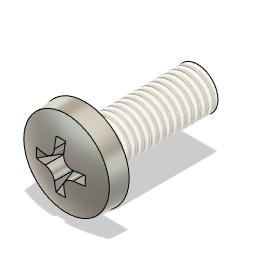
Pineapple case (Autodesk Fusion 360 archive; units mm, degrees)
design "Binding Head Screw JIS B 1111 - M3x8 Steel 4.6 Plain"
description: Binding Head Screw JIS B 1111 - M3x8
part number: BHS JIS B 1111 - M3x8 Steel 4.6 Plain
Autodesk Fusion 360 part; units mm, degrees
(part 1 of 2)
sketch "Sketch1" plane through (0, 0, 0) normal (0, 1, 0) x (1, 0, 0)
  line L0 (0, -1.9) -> (0, 8)
  line L1 (-3.15, 0) -> (-3.0363, -1.3)
  line L2 (-3.15, 0) -> (-1.299, 0)
  arc A0 (-3.0363, -1.3) -> (0, -1.9) centre (0, 6.0824) ccw
  line L3 (0, 8) -> (-1.5, 8)
  line L4 (-1.5, 8) -> (-1.5, 0.94)
  line L5 (-1.5, 0.94) -> (-1.299, 0.19)
  line L6 (-1.299, 0.19) -> (-1.299, 0)
  dimension "d13" = 5
  dimension "d14" = 6.3
  dimension "d18" = 3
  dimension "d23" = 15
  dimension "d53" = 1.9
  dimension "d55" = 7.06
  dimension "d56" = 8
  dimension "d57" = 7.81
  dimension "d60" = 1.3
  constraint vertical L0
  constraint coincident origin L0
  constraint horizontal L2
  constraint coincident origin L2
  constraint coincident L0 A0.end
  constraint coincident L0 A0.centre
  constraint coincident L0.start A0.end
  constraint perpendicular L0 L3
  constraint perpendicular L3 L4
  constraint vertical L6
  constraint coincident L2.end L6.end
  measures "d13" angle of L0 L1
  measures "d23" angle of L4 L5
  measures "d53" distance of L0.start L2
  measures "d55" distance of L3 L4.end
  measures "d56" distance of L2 L3
  measures "d57" distance of L3 L5.end
  measures "d60" distance of L1.end L2
revolve "Revolve1" add sketch "Sketch1" angle 360 about axis through (0, 0, 1.9) along (0, 0, -1) makes body 1
fillet "Fillet2" radius 0.1 1 edges at (-1.2111, 0.4698, 0) on bodies 1
ref_plane "WorkPlane1" through (0, 0, 1.9) normal (0, 0, 1) x (1, 0, 0)
sketch "Sketch2" plane through (0, 0, 1.9) normal (0, 0, 1) x (1, 0, 0)
  line L0 (-1.85, 0) -> (1.85, 0) construction
  line L1 (0, -1.85) -> (0, 1.85) construction
  line L2 (-0.331, 1.85) -> (0.331, 1.85)
  line L3 (0.331, 1.85) -> (0.331, 0.331)
  line L4 (0.331, 0.331) -> (1.85, 0.331)
  line L5 (1.85, 0.331) -> (1.85, -0.331)
  line L6 (1.85, -0.331) -> (0.331, -0.331)
  line L7 (0.331, -0.331) -> (0.331, -1.85)
  line L8 (0.331, -1.85) -> (-0.331, -1.85)
  line L9 (-0.331, -1.85) -> (-0.331, -0.331)
  line L10 (-0.331, -0.331) -> (-1.85, -0.331)
  line L11 (-1.85, -0.331) -> (-1.85, 0.331)
  line L12 (-1.85, 0.331) -> (-0.331, 0.331)
  line L13 (-0.331, 0.331) -> (-0.331, 1.85)
  dimension "d58" = 0.662
  dimension "d59" = 0.662
  dimension "d61" = 3.7
  dimension "d62" = 3.7
  constraint horizontal L0
  constraint vertical L1
  constraint midpoint L0 L1
  constraint midpoint origin L1
  constraint perpendicular L1 L2
  constraint perpendicular L2 L3
  constraint perpendicular L3 L4
  constraint perpendicular L0 L5
  constraint perpendicular L5 L6
  constraint perpendicular L0 L7
  constraint perpendicular L7 L8
  constraint perpendicular L8 L9
  constraint perpendicular L7 L10
  constraint perpendicular L10 L11
  constraint perpendicular L11 L12
  constraint vertical L13
  constraint coincident L9 L12.end
  constraint coincident L3.end L7
  constraint coincident L6 L9.end
  constraint coincident L4 L12.end
  constraint midpoint L0.end L5
  constraint midpoint L1.start L8
  constraint midpoint L1.end L2
  constraint midpoint L0.start L11
  measures "d58" distance of L10 L12
  measures "d59" distance of L3 L13
  measures "d61" distance of L2 L8
  measures "d62" distance of L5 L11
extrude "Extrude1" add sketch "Sketch2" against normal blind 1.53 separate body makes body 2
draft "Draft1" angle -30 neutral plane through (0, 0, 1.9) pull (0, 0, 1) 4 faces at (0.1103, -1.85, 1.39) (-0.1103, 1.85, 1.39) (-1.85, -0.1103, 1.39) (1.85, 0.1103, 1.39) on bodies 2
fillet "Fillet1" radius 0.662 4 edges at (0.331, -0.331, 1.135) (-0.331, -0.331, 1.135) (-0.331, 0.331, 1.135) (0.331, 0.331, 1.135) on bodies 2
combine "Combine1" operation cut target body 1 tool bodies 2
thread "Thread1" "ISO Metric profile 3.0 M3x0.5 M3x0.5 6g" major diameter 2.927 minor diameter 2.3555 pitch 0.5 angle 60 resizes the face on face at (-1.4925, -0.1494, -5.6467) on bodies 1
equation "adsk_nomdia = 3.00 mm"
equation "adsk_nomlen = 8.00 mm"
equation "adsk_headdia = 6.30 mm"
equation "adsk_baseh = 1.30 mm"
equation "adsk_phildia = 3.70 mm"
equation "adsk_midfillet = 0.10 mm"
equation "adsk_thrlen = 7.06 mm"
equation "adsk_phildepth = 1.53 mm"
equation "adsk_thrrun = 0.75 mm"
equation "adsk_thrang = 15.00 deg"
equation "adsk_headang = 5.00 deg"
equation "d13 = adsk_headang"
equation "d14 = adsk_headdia"
equation "adsk_ovalh = 0.60 mm"
equation "d18 = adsk_nomdia"
equation "d23 = adsk_thrang"
equation "d32 = adsk_baseh + adsk_ovalh"
equation "adsk_philwidth = 0.662 mm"
equation "d43 = -adsk_phildepth"
equation "d48 = adsk_philwidth"
equation "d52 = adsk_midfillet"
equation "d53 = adsk_baseh + adsk_ovalh"
equation "d55 = adsk_thrlen"
equation "d56 = adsk_nomlen"
equation "d57 = adsk_thrlen + adsk_thrrun"
equation "d58 = adsk_philwidth"
equation "d59 = adsk_philwidth"
equation "d60 = adsk_baseh"
equation "d61 = adsk_phildia"
equation "d62 = adsk_phildia"

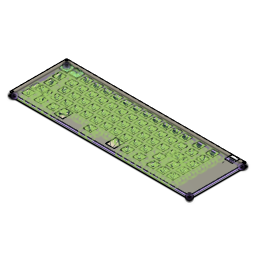
design "Pineappletopcover"
part number: 2025-06-25-20-34-07-285
Autodesk Fusion 360 part; units mm, degrees
sketch "Sketch1" plane through (0, 0, 0) normal (0, 0, 1) x (1, 0, 0)
sketch "Sketch2" plane through (0, 0, 0) normal (0, 0, 1) x (1, 0, 0)
  line L0 (-149.054719, 54.242084) -> (-136.054719, 54.242084)
  line L1 (-149.054719, 40.242084) -> (-136.054719, 40.242084)
  line L2 (-149.554719, 53.742084) -> (-149.554719, 40.742084)
  line L3 (-135.554719, 53.742084) -> (-135.554719, 40.742084)
  arc A0 (-149.054719, 54.242084) -> (-149.554719, 53.742084) centre (-149.054719, 53.742084) ccw
  arc A1 (-135.554719, 53.742084) -> (-136.054719, 54.242084) centre (-136.054719, 53.742084) ccw
  arc A2 (-149.554719, 40.742084) -> (-149.054719, 40.242084) centre (-149.054719, 40.742084) ccw
  arc A3 (-136.054719, 40.242084) -> (-135.554719, 40.742084) centre (-136.054719, 40.742084) ccw
  line L4 (-130.004719, 54.242084) -> (-117.004719, 54.242084)
  line L5 (-130.004719, 40.242084) -> (-117.004719, 40.242084)
  line L6 (-130.504719, 53.742084) -> (-130.504719, 40.742084)
  line L7 (-116.504719, 53.742084) -> (-116.504719, 40.742084)
  arc A4 (-130.004719, 54.242084) -> (-130.504719, 53.742084) centre (-130.004719, 53.742084) ccw
  arc A5 (-116.504719, 53.742084) -> (-117.004719, 54.242084) centre (-117.004719, 53.742084) ccw
  arc A6 (-130.504719, 40.742084) -> (-130.004719, 40.242084) centre (-130.004719, 40.742084) ccw
  arc A7 (-117.004719, 40.242084) -> (-116.504719, 40.742084) centre (-117.004719, 40.742084) ccw
  line L8 (-110.954719, 54.242084) -> (-97.954719, 54.242084)
  line L9 (-110.954719, 40.242084) -> (-97.954719, 40.242084)
  line L10 (-111.454719, 53.742084) -> (-111.454719, 40.742084)
  line L11 (-97.454719, 53.742084) -> (-97.454719, 40.742084)
  arc A8 (-110.954719, 54.242084) -> (-111.454719, 53.742084) centre (-110.954719, 53.742084) ccw
  arc A9 (-97.454719, 53.742084) -> (-97.954719, 54.242084) centre (-97.954719, 53.742084) ccw
  arc A10 (-111.454719, 40.742084) -> (-110.954719, 40.242084) centre (-110.954719, 40.742084) ccw
  arc A11 (-97.954719, 40.242084) -> (-97.454719, 40.742084) centre (-97.954719, 40.742084) ccw
  line L12 (-91.904719, 54.242084) -> (-78.904719, 54.242084)
  line L13 (-91.904719, 40.242084) -> (-78.904719, 40.242084)
  line L14 (-92.404719, 53.742084) -> (-92.404719, 40.742084)
  line L15 (-78.404719, 53.742084) -> (-78.404719, 40.742084)
  arc A12 (-91.904719, 54.242084) -> (-92.404719, 53.742084) centre (-91.904719, 53.742084) ccw
  arc A13 (-78.404719, 53.742084) -> (-78.904719, 54.242084) centre (-78.904719, 53.742084) ccw
  arc A14 (-92.404719, 40.742084) -> (-91.904719, 40.242084) centre (-91.904719, 40.742084) ccw
  arc A15 (-78.904719, 40.242084) -> (-78.404719, 40.742084) centre (-78.904719, 40.742084) ccw
  line L16 (-72.854719, 54.242084) -> (-59.854719, 54.242084)
  line L17 (-72.854719, 40.242084) -> (-59.854719, 40.242084)
  line L18 (-73.354719, 53.742084) -> (-73.354719, 40.742084)
  line L19 (-59.354719, 53.742084) -> (-59.354719, 40.742084)
  arc A16 (-72.854719, 54.242084) -> (-73.354719, 53.742084) centre (-72.854719, 53.742084) ccw
  arc A17 (-59.354719, 53.742084) -> (-59.854719, 54.242084) centre (-59.854719, 53.742084) ccw
  arc A18 (-73.354719, 40.742084) -> (-72.854719, 40.242084) centre (-72.854719, 40.742084) ccw
  arc A19 (-59.854719, 40.242084) -> (-59.354719, 40.742084) centre (-59.854719, 40.742084) ccw
  line L20 (-53.804719, 54.242084) -> (-40.804719, 54.242084)
  line L21 (-53.804719, 40.242084) -> (-40.804719, 40.242084)
  line L22 (-54.304719, 53.742084) -> (-54.304719, 40.742084)
  line L23 (-40.304719, 53.742084) -> (-40.304719, 40.742084)
  arc A20 (-53.804719, 54.242084) -> (-54.304719, 53.742084) centre (-53.804719, 53.742084) ccw
  arc A21 (-40.304719, 53.742084) -> (-40.804719, 54.242084) centre (-40.804719, 53.742084) ccw
  arc A22 (-54.304719, 40.742084) -> (-53.804719, 40.242084) centre (-53.804719, 40.742084) ccw
  arc A23 (-40.804719, 40.242084) -> (-40.304719, 40.742084) centre (-40.804719, 40.742084) ccw
  line L24 (-34.754719, 54.242084) -> (-21.754719, 54.242084)
  line L25 (-34.754719, 40.242084) -> (-21.754719, 40.242084)
  line L26 (-35.254719, 53.742084) -> (-35.254719, 40.742084)
  line L27 (-21.254719, 53.742084) -> (-21.254719, 40.742084)
  arc A24 (-34.754719, 54.242084) -> (-35.254719, 53.742084) centre (-34.754719, 53.742084) ccw
  arc A25 (-21.254719, 53.742084) -> (-21.754719, 54.242084) centre (-21.754719, 53.742084) ccw
  arc A26 (-35.254719, 40.742084) -> (-34.754719, 40.242084) centre (-34.754719, 40.742084) ccw
  arc A27 (-21.754719, 40.242084) -> (-21.254719, 40.742084) centre (-21.754719, 40.742084) ccw
  line L28 (-15.704719, 54.242084) -> (-2.704719, 54.242084)
  line L29 (-15.704719, 40.242084) -> (-2.704719, 40.242084)
  line L30 (-16.204719, 53.742084) -> (-16.204719, 40.742084)
  line L31 (-2.204719, 53.742084) -> (-2.204719, 40.742084)
  arc A28 (-15.704719, 54.242084) -> (-16.204719, 53.742084) centre (-15.704719, 53.742084) ccw
  arc A29 (-2.204719, 53.742084) -> (-2.704719, 54.242084) centre (-2.704719, 53.742084) ccw
  arc A30 (-16.204719, 40.742084) -> (-15.704719, 40.242084) centre (-15.704719, 40.742084) ccw
  arc A31 (-2.704719, 40.242084) -> (-2.204719, 40.742084) centre (-2.704719, 40.742084) ccw
  line L32 (3.345281, 54.242084) -> (16.345281, 54.242084)
  line L33 (3.345281, 40.242084) -> (16.345281, 40.242084)
  line L34 (2.845281, 53.742084) -> (2.845281, 40.742084)
  line L35 (16.845281, 53.742084) -> (16.845281, 40.742084)
  arc A32 (3.345281, 54.242084) -> (2.845281, 53.742084) centre (3.345281, 53.742084) ccw
  arc A33 (16.845281, 53.742084) -> (16.345281, 54.242084) centre (16.345281, 53.742084) ccw
  arc A34 (2.845281, 40.742084) -> (3.345281, 40.242084) centre (3.345281, 40.742084) ccw
  arc A35 (16.345281, 40.242084) -> (16.845281, 40.742084) centre (16.345281, 40.742084) ccw
  line L36 (22.395281, 54.242084) -> (35.395281, 54.242084)
  line L37 (22.395281, 40.242084) -> (35.395281, 40.242084)
  line L38 (21.895281, 53.742084) -> (21.895281, 40.742084)
  line L39 (35.895281, 53.742084) -> (35.895281, 40.742084)
  arc A36 (22.395281, 54.242084) -> (21.895281, 53.742084) centre (22.395281, 53.742084) ccw
  arc A37 (35.895281, 53.742084) -> (35.395281, 54.242084) centre (35.395281, 53.742084) ccw
  arc A38 (21.895281, 40.742084) -> (22.395281, 40.242084) centre (22.395281, 40.742084) ccw
  arc A39 (35.395281, 40.242084) -> (35.895281, 40.742084) centre (35.395281, 40.742084) ccw
  line L40 (41.445281, 54.242084) -> (54.445281, 54.242084)
  line L41 (41.445281, 40.242084) -> (54.445281, 40.242084)
  line L42 (40.945281, 53.742084) -> (40.945281, 40.742084)
  line L43 (54.945281, 53.742084) -> (54.945281, 40.742084)
  arc A40 (41.445281, 54.242084) -> (40.945281, 53.742084) centre (41.445281, 53.742084) ccw
  arc A41 (54.945281, 53.742084) -> (54.445281, 54.242084) centre (54.445281, 53.742084) ccw
  arc A42 (40.945281, 40.742084) -> (41.445281, 40.242084) centre (41.445281, 40.742084) ccw
  arc A43 (54.445281, 40.242084) -> (54.945281, 40.742084) centre (54.445281, 40.742084) ccw
  line L44 (60.495281, 54.242084) -> (73.495281, 54.242084)
  line L45 (60.495281, 40.242084) -> (73.495281, 40.242084)
  line L46 (59.995281, 53.742084) -> (59.995281, 40.742084)
  line L47 (73.995281, 53.742084) -> (73.995281, 40.742084)
  arc A44 (60.495281, 54.242084) -> (59.995281, 53.742084) centre (60.495281, 53.742084) ccw
  arc A45 (73.995281, 53.742084) -> (73.495281, 54.242084) centre (73.495281, 53.742084) ccw
  arc A46 (59.995281, 40.742084) -> (60.495281, 40.242084) centre (60.495281, 40.742084) ccw
  arc A47 (73.495281, 40.242084) -> (73.995281, 40.742084) centre (73.495281, 40.742084) ccw
  line L48 (79.545281, 54.242084) -> (92.545281, 54.242084)
  line L49 (79.545281, 40.242084) -> (92.545281, 40.242084)
  line L50 (79.045281, 53.742084) -> (79.045281, 40.742084)
  line L51 (93.045281, 53.742084) -> (93.045281, 40.742084)
  arc A48 (79.545281, 54.242084) -> (79.045281, 53.742084) centre (79.545281, 53.742084) ccw
  arc A49 (93.045281, 53.742084) -> (92.545281, 54.242084) centre (92.545281, 53.742084) ccw
  arc A50 (79.045281, 40.742084) -> (79.545281, 40.242084) centre (79.545281, 40.742084) ccw
  arc A51 (92.545281, 40.242084) -> (93.045281, 40.742084) centre (92.545281, 40.742084) ccw
  line L52 (105.739031, 54.242084) -> (118.739031, 54.242084)
  line L53 (105.739031, 40.242084) -> (118.739031, 40.242084)
  line L54 (105.239031, 53.742084) -> (105.239031, 40.742084)
  line L55 (119.239031, 53.742084) -> (119.239031, 40.742084)
  arc A52 (105.739031, 54.242084) -> (105.239031, 53.742084) centre (105.739031, 53.742084) ccw
  arc A53 (119.239031, 53.742084) -> (118.739031, 54.242084) centre (118.739031, 53.742084) ccw
  arc A54 (105.239031, 40.742084) -> (105.739031, 40.242084) centre (105.739031, 40.742084) ccw
  arc A55 (118.739031, 40.242084) -> (119.239031, 40.742084) centre (118.739031, 40.742084) ccw
  line L56 (131.932781, 54.242084) -> (144.932781, 54.242084)
  line L57 (131.932781, 40.242084) -> (144.932781, 40.242084)
  line L58 (131.432781, 53.742084) -> (131.432781, 40.742084)
  line L59 (145.432781, 53.742084) -> (145.432781, 40.742084)
  arc A56 (131.932781, 54.242084) -> (131.432781, 53.742084) centre (131.932781, 53.742084) ccw
  arc A57 (145.432781, 53.742084) -> (144.932781, 54.242084) centre (144.932781, 53.742084) ccw
  arc A58 (131.432781, 40.742084) -> (131.932781, 40.242084) centre (131.932781, 40.742084) ccw
  arc A59 (144.932781, 40.242084) -> (145.432781, 40.742084) centre (144.932781, 40.742084) ccw
  line L60 (-144.292219, 35.192084) -> (-131.292219, 35.192084)
  line L61 (-144.292219, 21.192084) -> (-131.292219, 21.192084)
  line L62 (-144.792219, 34.692084) -> (-144.792219, 21.692084)
  line L63 (-130.792219, 34.692084) -> (-130.792219, 21.692084)
  arc A60 (-144.292219, 35.192084) -> (-144.792219, 34.692084) centre (-144.292219, 34.692084) ccw
  arc A61 (-130.792219, 34.692084) -> (-131.292219, 35.192084) centre (-131.292219, 34.692084) ccw
  arc A62 (-144.792219, 21.692084) -> (-144.292219, 21.192084) centre (-144.292219, 21.692084) ccw
  arc A63 (-131.292219, 21.192084) -> (-130.792219, 21.692084) centre (-131.292219, 21.692084) ccw
  line L64 (-120.479719, 35.192084) -> (-107.479719, 35.192084)
  line L65 (-120.479719, 21.192084) -> (-107.479719, 21.192084)
  line L66 (-120.979719, 34.692084) -> (-120.979719, 21.692084)
  line L67 (-106.979719, 34.692084) -> (-106.979719, 21.692084)
  arc A64 (-120.479719, 35.192084) -> (-120.979719, 34.692084) centre (-120.479719, 34.692084) ccw
  arc A65 (-106.979719, 34.692084) -> (-107.479719, 35.192084) centre (-107.479719, 34.692084) ccw
  arc A66 (-120.979719, 21.692084) -> (-120.479719, 21.192084) centre (-120.479719, 21.692084) ccw
  arc A67 (-107.479719, 21.192084) -> (-106.979719, 21.692084) centre (-107.479719, 21.692084) ccw
  line L68 (-101.429719, 35.192084) -> (-88.429719, 35.192084)
  line L69 (-101.429719, 21.192084) -> (-88.429719, 21.192084)
  line L70 (-101.929719, 34.692084) -> (-101.929719, 21.692084)
  line L71 (-87.929719, 34.692084) -> (-87.929719, 21.692084)
  arc A68 (-101.429719, 35.192084) -> (-101.929719, 34.692084) centre (-101.429719, 34.692084) ccw
  arc A69 (-87.929719, 34.692084) -> (-88.429719, 35.192084) centre (-88.429719, 34.692084) ccw
  arc A70 (-101.929719, 21.692084) -> (-101.429719, 21.192084) centre (-101.429719, 21.692084) ccw
  arc A71 (-88.429719, 21.192084) -> (-87.929719, 21.692084) centre (-88.429719, 21.692084) ccw
  line L72 (-82.379719, 35.192084) -> (-69.379719, 35.192084)
  line L73 (-82.379719, 21.192084) -> (-69.379719, 21.192084)
  line L74 (-82.879719, 34.692084) -> (-82.879719, 21.692084)
  line L75 (-68.879719, 34.692084) -> (-68.879719, 21.692084)
  arc A72 (-82.379719, 35.192084) -> (-82.879719, 34.692084) centre (-82.379719, 34.692084) ccw
  arc A73 (-68.879719, 34.692084) -> (-69.379719, 35.192084) centre (-69.379719, 34.692084) ccw
  arc A74 (-82.879719, 21.692084) -> (-82.379719, 21.192084) centre (-82.379719, 21.692084) ccw
  arc A75 (-69.379719, 21.192084) -> (-68.879719, 21.692084) centre (-69.379719, 21.692084) ccw
  line L76 (-63.329719, 35.192084) -> (-50.329719, 35.192084)
  line L77 (-63.329719, 21.192084) -> (-50.329719, 21.192084)
  line L78 (-63.829719, 34.692084) -> (-63.829719, 21.692084)
  line L79 (-49.829719, 34.692084) -> (-49.829719, 21.692084)
  arc A76 (-63.329719, 35.192084) -> (-63.829719, 34.692084) centre (-63.329719, 34.692084) ccw
  arc A77 (-49.829719, 34.692084) -> (-50.329719, 35.192084) centre (-50.329719, 34.692084) ccw
  arc A78 (-63.829719, 21.692084) -> (-63.329719, 21.192084) centre (-63.329719, 21.692084) ccw
  arc A79 (-50.329719, 21.192084) -> (-49.829719, 21.692084) centre (-50.329719, 21.692084) ccw
  line L80 (-44.279719, 35.192084) -> (-31.279719, 35.192084)
  line L81 (-44.279719, 21.192084) -> (-31.279719, 21.192084)
  line L82 (-44.779719, 34.692084) -> (-44.779719, 21.692084)
  line L83 (-30.779719, 34.692084) -> (-30.779719, 21.692084)
  arc A80 (-44.279719, 35.192084) -> (-44.779719, 34.692084) centre (-44.279719, 34.692084) ccw
  arc A81 (-30.779719, 34.692084) -> (-31.279719, 35.192084) centre (-31.279719, 34.692084) ccw
  arc A82 (-44.779719, 21.692084) -> (-44.279719, 21.192084) centre (-44.279719, 21.692084) ccw
  arc A83 (-31.279719, 21.192084) -> (-30.779719, 21.692084) centre (-31.279719, 21.692084) ccw
  line L84 (-25.229719, 35.192084) -> (-12.229719, 35.192084)
  line L85 (-25.229719, 21.192084) -> (-12.229719, 21.192084)
  line L86 (-25.729719, 34.692084) -> (-25.729719, 21.692084)
  line L87 (-11.729719, 34.692084) -> (-11.729719, 21.692084)
  arc A84 (-25.229719, 35.192084) -> (-25.729719, 34.692084) centre (-25.229719, 34.692084) ccw
  arc A85 (-11.729719, 34.692084) -> (-12.229719, 35.192084) centre (-12.229719, 34.692084) ccw
  arc A86 (-25.729719, 21.692084) -> (-25.229719, 21.192084) centre (-25.229719, 21.692084) ccw
  arc A87 (-12.229719, 21.192084) -> (-11.729719, 21.692084) centre (-12.229719, 21.692084) ccw
  line L88 (-6.179719, 35.192084) -> (6.820281, 35.192084)
  line L89 (-6.179719, 21.192084) -> (6.820281, 21.192084)
  line L90 (-6.679719, 34.692084) -> (-6.679719, 21.692084)
  line L91 (7.320281, 34.692084) -> (7.320281, 21.692084)
  arc A88 (-6.179719, 35.192084) -> (-6.679719, 34.692084) centre (-6.179719, 34.692084) ccw
  arc A89 (7.320281, 34.692084) -> (6.820281, 35.192084) centre (6.820281, 34.692084) ccw
  arc A90 (-6.679719, 21.692084) -> (-6.179719, 21.192084) centre (-6.179719, 21.692084) ccw
  arc A91 (6.820281, 21.192084) -> (7.320281, 21.692084) centre (6.820281, 21.692084) ccw
  line L92 (12.870281, 35.192084) -> (25.870281, 35.192084)
  line L93 (12.870281, 21.192084) -> (25.870281, 21.192084)
  line L94 (12.370281, 34.692084) -> (12.370281, 21.692084)
  line L95 (26.370281, 34.692084) -> (26.370281, 21.692084)
  arc A92 (12.870281, 35.192084) -> (12.370281, 34.692084) centre (12.870281, 34.692084) ccw
  arc A93 (26.370281, 34.692084) -> (25.870281, 35.192084) centre (25.870281, 34.692084) ccw
  arc A94 (12.370281, 21.692084) -> (12.870281, 21.192084) centre (12.870281, 21.692084) ccw
  arc A95 (25.870281, 21.192084) -> (26.370281, 21.692084) centre (25.870281, 21.692084) ccw
  line L96 (31.920281, 35.192084) -> (44.920281, 35.192084)
  line L97 (31.920281, 21.192084) -> (44.920281, 21.192084)
  line L98 (31.420281, 34.692084) -> (31.420281, 21.692084)
  line L99 (45.420281, 34.692084) -> (45.420281, 21.692084)
  arc A96 (31.920281, 35.192084) -> (31.420281, 34.692084) centre (31.920281, 34.692084) ccw
  arc A97 (45.420281, 34.692084) -> (44.920281, 35.192084) centre (44.920281, 34.692084) ccw
  arc A98 (31.420281, 21.692084) -> (31.920281, 21.192084) centre (31.920281, 21.692084) ccw
  arc A99 (44.920281, 21.192084) -> (45.420281, 21.692084) centre (44.920281, 21.692084) ccw
  line L100 (50.970281, 35.192084) -> (63.970281, 35.192084)
  line L101 (50.970281, 21.192084) -> (63.970281, 21.192084)
  line L102 (50.470281, 34.692084) -> (50.470281, 21.692084)
  line L103 (64.470281, 34.692084) -> (64.470281, 21.692084)
  arc A100 (50.970281, 35.192084) -> (50.470281, 34.692084) centre (50.970281, 34.692084) ccw
  arc A101 (64.470281, 34.692084) -> (63.970281, 35.192084) centre (63.970281, 34.692084) ccw
  arc A102 (50.470281, 21.692084) -> (50.970281, 21.192084) centre (50.970281, 21.692084) ccw
  arc A103 (63.970281, 21.192084) -> (64.470281, 21.692084) centre (63.970281, 21.692084) ccw
  line L104 (70.020281, 35.192084) -> (83.020281, 35.192084)
  line L105 (70.020281, 21.192084) -> (83.020281, 21.192084)
  line L106 (69.520281, 34.692084) -> (69.520281, 21.692084)
  line L107 (83.520281, 34.692084) -> (83.520281, 21.692084)
  arc A104 (70.020281, 35.192084) -> (69.520281, 34.692084) centre (70.020281, 34.692084) ccw
  arc A105 (83.520281, 34.692084) -> (83.020281, 35.192084) centre (83.020281, 34.692084) ccw
  arc A106 (69.520281, 21.692084) -> (70.020281, 21.192084) centre (70.020281, 21.692084) ccw
  arc A107 (83.020281, 21.192084) -> (83.520281, 21.692084) centre (83.020281, 21.692084) ccw
  line L108 (89.070281, 35.192084) -> (102.070281, 35.192084)
  line L109 (89.070281, 21.192084) -> (102.070281, 21.192084)
  line L110 (88.570281, 34.692084) -> (88.570281, 21.692084)
  line L111 (102.570281, 34.692084) -> (102.570281, 21.692084)
  arc A108 (89.070281, 35.192084) -> (88.570281, 34.692084) centre (89.070281, 34.692084) ccw
  arc A109 (102.570281, 34.692084) -> (102.070281, 35.192084) centre (102.070281, 34.692084) ccw
  arc A110 (88.570281, 21.692084) -> (89.070281, 21.192084) centre (89.070281, 21.692084) ccw
  arc A111 (102.070281, 21.192084) -> (102.570281, 21.692084) centre (102.070281, 21.692084) ccw
  line L112 (110.501531, 35.192084) -> (123.501531, 35.192084)
  line L113 (110.501531, 21.192084) -> (123.501531, 21.192084)
  line L114 (110.001531, 34.692084) -> (110.001531, 21.692084)
  line L115 (124.001531, 34.692084) -> (124.001531, 21.692084)
  arc A112 (110.501531, 35.192084) -> (110.001531, 34.692084) centre (110.501531, 34.692084) ccw
  arc A113 (124.001531, 34.692084) -> (123.501531, 35.192084) centre (123.501531, 34.692084) ccw
  arc A114 (110.001531, 21.692084) -> (110.501531, 21.192084) centre (110.501531, 21.692084) ccw
  arc A115 (123.501531, 21.192084) -> (124.001531, 21.692084) centre (123.501531, 21.692084) ccw
  line L116 (131.932781, 35.192084) -> (144.932781, 35.192084)
  line L117 (131.932781, 21.192084) -> (144.932781, 21.192084)
  line L118 (131.432781, 34.692084) -> (131.432781, 21.692084)
  line L119 (145.432781, 34.692084) -> (145.432781, 21.692084)
  arc A116 (131.932781, 35.192084) -> (131.432781, 34.692084) centre (131.932781, 34.692084) ccw
  arc A117 (145.432781, 34.692084) -> (144.932781, 35.192084) centre (144.932781, 34.692084) ccw
  arc A118 (131.432781, 21.692084) -> (131.932781, 21.192084) centre (131.932781, 21.692084) ccw
  arc A119 (144.932781, 21.192084) -> (145.432781, 21.692084) centre (144.932781, 21.692084) ccw
  line L120 (-141.910969, 16.142084) -> (-128.910969, 16.142084)
  line L121 (-141.910969, 2.142084) -> (-128.910969, 2.142084)
  line L122 (-142.410969, 15.642084) -> (-142.410969, 2.642084)
  line L123 (-128.410969, 15.642084) -> (-128.410969, 2.642084)
  arc A120 (-141.910969, 16.142084) -> (-142.410969, 15.642084) centre (-141.910969, 15.642084) ccw
  arc A121 (-128.410969, 15.642084) -> (-128.910969, 16.142084) centre (-128.910969, 15.642084) ccw
  arc A122 (-142.410969, 2.642084) -> (-141.910969, 2.142084) centre (-141.910969, 2.642084) ccw
  arc A123 (-128.910969, 2.142084) -> (-128.410969, 2.642084) centre (-128.910969, 2.642084) ccw
  line L124 (-115.717219, 16.142084) -> (-102.717219, 16.142084)
  line L125 (-115.717219, 2.142084) -> (-102.717219, 2.142084)
  line L126 (-116.217219, 15.642084) -> (-116.217219, 2.642084)
  line L127 (-102.217219, 15.642084) -> (-102.217219, 2.642084)
  arc A124 (-115.717219, 16.142084) -> (-116.217219, 15.642084) centre (-115.717219, 15.642084) ccw
  arc A125 (-102.217219, 15.642084) -> (-102.717219, 16.142084) centre (-102.717219, 15.642084) ccw
  arc A126 (-116.217219, 2.642084) -> (-115.717219, 2.142084) centre (-115.717219, 2.642084) ccw
  arc A127 (-102.717219, 2.142084) -> (-102.217219, 2.642084) centre (-102.717219, 2.642084) ccw
  line L128 (-96.667219, 16.142084) -> (-83.667219, 16.142084)
  line L129 (-96.667219, 2.142084) -> (-83.667219, 2.142084)
  line L130 (-97.167219, 15.642084) -> (-97.167219, 2.642084)
  line L131 (-83.167219, 15.642084) -> (-83.167219, 2.642084)
  arc A128 (-96.667219, 16.142084) -> (-97.167219, 15.642084) centre (-96.667219, 15.642084) ccw
  arc A129 (-83.167219, 15.642084) -> (-83.667219, 16.142084) centre (-83.667219, 15.642084) ccw
  arc A130 (-97.167219, 2.642084) -> (-96.667219, 2.142084) centre (-96.667219, 2.642084) ccw
  arc A131 (-83.667219, 2.142084) -> (-83.167219, 2.642084) centre (-83.667219, 2.642084) ccw
  line L132 (-77.617219, 16.142084) -> (-64.617219, 16.142084)
  line L133 (-77.617219, 2.142084) -> (-64.617219, 2.142084)
  line L134 (-78.117219, 15.642084) -> (-78.117219, 2.642084)
  line L135 (-64.117219, 15.642084) -> (-64.117219, 2.642084)
  arc A132 (-77.617219, 16.142084) -> (-78.117219, 15.642084) centre (-77.617219, 15.642084) ccw
  arc A133 (-64.117219, 15.642084) -> (-64.617219, 16.142084) centre (-64.617219, 15.642084) ccw
  arc A134 (-78.117219, 2.642084) -> (-77.617219, 2.142084) centre (-77.617219, 2.642084) ccw
  arc A135 (-64.617219, 2.142084) -> (-64.117219, 2.642084) centre (-64.617219, 2.642084) ccw
  line L136 (-58.567219, 16.142084) -> (-45.567219, 16.142084)
  line L137 (-58.567219, 2.142084) -> (-45.567219, 2.142084)
  line L138 (-59.067219, 15.642084) -> (-59.067219, 2.642084)
  line L139 (-45.067219, 15.642084) -> (-45.067219, 2.642084)
  arc A136 (-58.567219, 16.142084) -> (-59.067219, 15.642084) centre (-58.567219, 15.642084) ccw
  arc A137 (-45.067219, 15.642084) -> (-45.567219, 16.142084) centre (-45.567219, 15.642084) ccw
  arc A138 (-59.067219, 2.642084) -> (-58.567219, 2.142084) centre (-58.567219, 2.642084) ccw
  arc A139 (-45.567219, 2.142084) -> (-45.067219, 2.642084) centre (-45.567219, 2.642084) ccw
  line L140 (-39.517219, 16.142084) -> (-26.517219, 16.142084)
  line L141 (-39.517219, 2.142084) -> (-26.517219, 2.142084)
  line L142 (-40.017219, 15.642084) -> (-40.017219, 2.642084)
  line L143 (-26.017219, 15.642084) -> (-26.017219, 2.642084)
  arc A140 (-39.517219, 16.142084) -> (-40.017219, 15.642084) centre (-39.517219, 15.642084) ccw
  arc A141 (-26.017219, 15.642084) -> (-26.517219, 16.142084) centre (-26.517219, 15.642084) ccw
  arc A142 (-40.017219, 2.642084) -> (-39.517219, 2.142084) centre (-39.517219, 2.642084) ccw
  arc A143 (-26.517219, 2.142084) -> (-26.017219, 2.642084) centre (-26.517219, 2.642084) ccw
  line L144 (-20.467219, 16.142084) -> (-7.467219, 16.142084)
  line L145 (-20.467219, 2.142084) -> (-7.467219, 2.142084)
  line L146 (-20.967219, 15.642084) -> (-20.967219, 2.642084)
  line L147 (-6.967219, 15.642084) -> (-6.967219, 2.642084)
  arc A144 (-20.467219, 16.142084) -> (-20.967219, 15.642084) centre (-20.467219, 15.642084) ccw
  arc A145 (-6.967219, 15.642084) -> (-7.467219, 16.142084) centre (-7.467219, 15.642084) ccw
  arc A146 (-20.967219, 2.642084) -> (-20.467219, 2.142084) centre (-20.467219, 2.642084) ccw
  arc A147 (-7.467219, 2.142084) -> (-6.967219, 2.642084) centre (-7.467219, 2.642084) ccw
  line L148 (-1.417219, 16.142084) -> (11.582781, 16.142084)
  line L149 (-1.417219, 2.142084) -> (11.582781, 2.142084)
  line L150 (-1.917219, 15.642084) -> (-1.917219, 2.642084)
  line L151 (12.082781, 15.642084) -> (12.082781, 2.642084)
  arc A148 (-1.417219, 16.142084) -> (-1.917219, 15.642084) centre (-1.417219, 15.642084) ccw
  arc A149 (12.082781, 15.642084) -> (11.582781, 16.142084) centre (11.582781, 15.642084) ccw
  arc A150 (-1.917219, 2.642084) -> (-1.417219, 2.142084) centre (-1.417219, 2.642084) ccw
  arc A151 (11.582781, 2.142084) -> (12.082781, 2.642084) centre (11.582781, 2.642084) ccw
  line L152 (17.632781, 16.142084) -> (30.632781, 16.142084)
  line L153 (17.632781, 2.142084) -> (30.632781, 2.142084)
  line L154 (17.132781, 15.642084) -> (17.132781, 2.642084)
  line L155 (31.132781, 15.642084) -> (31.132781, 2.642084)
  arc A152 (17.632781, 16.142084) -> (17.132781, 15.642084) centre (17.632781, 15.642084) ccw
  arc A153 (31.132781, 15.642084) -> (30.632781, 16.142084) centre (30.632781, 15.642084) ccw
  arc A154 (17.132781, 2.642084) -> (17.632781, 2.142084) centre (17.632781, 2.642084) ccw
  arc A155 (30.632781, 2.142084) -> (31.132781, 2.642084) centre (30.632781, 2.642084) ccw
  line L156 (36.682781, 16.142084) -> (49.682781, 16.142084)
  line L157 (36.682781, 2.142084) -> (49.682781, 2.142084)
  line L158 (36.182781, 15.642084) -> (36.182781, 2.642084)
  line L159 (50.182781, 15.642084) -> (50.182781, 2.642084)
  arc A156 (36.682781, 16.142084) -> (36.182781, 15.642084) centre (36.682781, 15.642084) ccw
  arc A157 (50.182781, 15.642084) -> (49.682781, 16.142084) centre (49.682781, 15.642084) ccw
  arc A158 (36.182781, 2.642084) -> (36.682781, 2.142084) centre (36.682781, 2.642084) ccw
  arc A159 (49.682781, 2.142084) -> (50.182781, 2.642084) centre (49.682781, 2.642084) ccw
  line L160 (55.732781, 16.142084) -> (68.732781, 16.142084)
  line L161 (55.732781, 2.142084) -> (68.732781, 2.142084)
  line L162 (55.232781, 15.642084) -> (55.232781, 2.642084)
  line L163 (69.232781, 15.642084) -> (69.232781, 2.642084)
  arc A160 (55.732781, 16.142084) -> (55.232781, 15.642084) centre (55.732781, 15.642084) ccw
  arc A161 (69.232781, 15.642084) -> (68.732781, 16.142084) centre (68.732781, 15.642084) ccw
  arc A162 (55.232781, 2.642084) -> (55.732781, 2.142084) centre (55.732781, 2.642084) ccw
  arc A163 (68.732781, 2.142084) -> (69.232781, 2.642084) centre (68.732781, 2.642084) ccw
  line L164 (74.782781, 16.142084) -> (87.782781, 16.142084)
  line L165 (74.782781, 2.142084) -> (87.782781, 2.142084)
  line L166 (74.282781, 15.642084) -> (74.282781, 2.642084)
  line L167 (88.282781, 15.642084) -> (88.282781, 2.642084)
  arc A164 (74.782781, 16.142084) -> (74.282781, 15.642084) centre (74.782781, 15.642084) ccw
  arc A165 (88.282781, 15.642084) -> (87.782781, 16.142084) centre (87.782781, 15.642084) ccw
  arc A166 (74.282781, 2.642084) -> (74.782781, 2.142084) centre (74.782781, 2.642084) ccw
  arc A167 (87.782781, 2.142084) -> (88.282781, 2.642084) centre (87.782781, 2.642084) ccw
  line L168 (103.357781, 16.142084) -> (116.357781, 16.142084)
  line L169 (103.357781, 2.142084) -> (116.357781, 2.142084)
  line L170 (102.857781, 15.642084) -> (102.857781, 2.642084)
  line L171 (116.857781, 15.642084) -> (116.857781, 2.642084)
  arc A168 (103.357781, 16.142084) -> (102.857781, 15.642084) centre (103.357781, 15.642084) ccw
  arc A169 (116.857781, 15.642084) -> (116.357781, 16.142084) centre (116.357781, 15.642084) ccw
  arc A170 (102.857781, 2.642084) -> (103.357781, 2.142084) centre (103.357781, 2.642084) ccw
  arc A171 (116.357781, 2.142084) -> (116.857781, 2.642084) centre (116.357781, 2.642084) ccw
  line L172 (94.919781, 15.142084) -> (100.919781, 15.142084)
  line L173 (94.919781, 0.142084) -> (100.919781, 0.142084)
  line L174 (94.419781, 14.642084) -> (94.419781, 0.642084)
  line L175 (101.419781, 14.642084) -> (101.419781, 0.642084)
  arc A172 (94.919781, 15.142084) -> (94.419781, 14.642084) centre (94.919781, 14.642084) ccw
  arc A173 (101.419781, 14.642084) -> (100.919781, 15.142084) centre (100.919781, 14.642084) ccw
  arc A174 (94.419781, 0.642084) -> (94.919781, 0.142084) centre (94.919781, 0.642084) ccw
  arc A175 (100.919781, 0.142084) -> (101.419781, 0.642084) centre (100.919781, 0.642084) ccw
  line L176 (118.795781, 15.142084) -> (124.795781, 15.142084)
  line L177 (118.795781, 0.142084) -> (124.795781, 0.142084)
  line L178 (118.295781, 14.642084) -> (118.295781, 0.642084)
  line L179 (125.295781, 14.642084) -> (125.295781, 0.642084)
  arc A176 (118.795781, 15.142084) -> (118.295781, 14.642084) centre (118.795781, 14.642084) ccw
  arc A177 (125.295781, 14.642084) -> (124.795781, 15.142084) centre (124.795781, 14.642084) ccw
  arc A178 (118.295781, 0.642084) -> (118.795781, 0.142084) centre (118.795781, 0.642084) ccw
  arc A179 (124.795781, 0.142084) -> (125.295781, 0.642084) centre (124.795781, 0.642084) ccw
  line L180 (131.932781, 16.142084) -> (144.932781, 16.142084)
  line L181 (131.932781, 2.142084) -> (144.932781, 2.142084)
  line L182 (131.432781, 15.642084) -> (131.432781, 2.642084)
  line L183 (145.432781, 15.642084) -> (145.432781, 2.642084)
  arc A180 (131.932781, 16.142084) -> (131.432781, 15.642084) centre (131.932781, 15.642084) ccw
  arc A181 (145.432781, 15.642084) -> (144.932781, 16.142084) centre (144.932781, 15.642084) ccw
  arc A182 (131.432781, 2.642084) -> (131.932781, 2.142084) centre (131.932781, 2.642084) ccw
  arc A183 (144.932781, 2.142084) -> (145.432781, 2.642084) centre (144.932781, 2.642084) ccw
  line L184 (-139.529719, -2.907916) -> (-126.529719, -2.907916)
  line L185 (-139.529719, -16.907916) -> (-126.529719, -16.907916)
  line L186 (-140.029719, -3.407916) -> (-140.029719, -16.407916)
  line L187 (-126.029719, -3.407916) -> (-126.029719, -16.407916)
  arc A184 (-139.529719, -2.907916) -> (-140.029719, -3.407916) centre (-139.529719, -3.407916) ccw
  arc A185 (-126.029719, -3.407916) -> (-126.529719, -2.907916) centre (-126.529719, -3.407916) ccw
  arc A186 (-140.029719, -16.407916) -> (-139.529719, -16.907916) centre (-139.529719, -16.407916) ccw
  arc A187 (-126.529719, -16.907916) -> (-126.029719, -16.407916) centre (-126.529719, -16.407916) ccw
  line L188 (-147.967719, -3.907916) -> (-141.967719, -3.907916)
  line L189 (-147.967719, -18.907916) -> (-141.967719, -18.907916)
  line L190 (-148.467719, -4.407916) -> (-148.467719, -18.407916)
  line L191 (-141.467719, -4.407916) -> (-141.467719, -18.407916)
  arc A188 (-147.967719, -3.907916) -> (-148.467719, -4.407916) centre (-147.967719, -4.407916) ccw
  arc A189 (-141.467719, -4.407916) -> (-141.967719, -3.907916) centre (-141.967719, -4.407916) ccw
  arc A190 (-148.467719, -18.407916) -> (-147.967719, -18.907916) centre (-147.967719, -18.407916) ccw
  arc A191 (-141.967719, -18.907916) -> (-141.467719, -18.407916) centre (-141.967719, -18.407916) ccw
  line L192 (-124.091719, -3.907916) -> (-118.091719, -3.907916)
  line L193 (-124.091719, -18.907916) -> (-118.091719, -18.907916)
  line L194 (-124.591719, -4.407916) -> (-124.591719, -18.407916)
  line L195 (-117.591719, -4.407916) -> (-117.591719, -18.407916)
  arc A192 (-124.091719, -3.907916) -> (-124.591719, -4.407916) centre (-124.091719, -4.407916) ccw
  arc A193 (-117.591719, -4.407916) -> (-118.091719, -3.907916) centre (-118.091719, -4.407916) ccw
  arc A194 (-124.591719, -18.407916) -> (-124.091719, -18.907916) centre (-124.091719, -18.407916) ccw
  arc A195 (-118.091719, -18.907916) -> (-117.591719, -18.407916) centre (-118.091719, -18.407916) ccw
  line L196 (-110.954719, -2.907916) -> (-97.954719, -2.907916)
  line L197 (-110.954719, -16.907916) -> (-97.954719, -16.907916)
  line L198 (-111.454719, -3.407916) -> (-111.454719, -16.407916)
  line L199 (-97.454719, -3.407916) -> (-97.454719, -16.407916)
  arc A196 (-110.954719, -2.907916) -> (-111.454719, -3.407916) centre (-110.954719, -3.407916) ccw
  arc A197 (-97.454719, -3.407916) -> (-97.954719, -2.907916) centre (-97.954719, -3.407916) ccw
  arc A198 (-111.454719, -16.407916) -> (-110.954719, -16.907916) centre (-110.954719, -16.407916) ccw
  arc A199 (-97.954719, -16.907916) -> (-97.454719, -16.407916) centre (-97.954719, -16.407916) ccw
  line L200 (-91.904719, -2.907916) -> (-78.904719, -2.907916)
  line L201 (-91.904719, -16.907916) -> (-78.904719, -16.907916)
  line L202 (-92.404719, -3.407916) -> (-92.404719, -16.407916)
  line L203 (-78.404719, -3.407916) -> (-78.404719, -16.407916)
  arc A200 (-91.904719, -2.907916) -> (-92.404719, -3.407916) centre (-91.904719, -3.407916) ccw
  arc A201 (-78.404719, -3.407916) -> (-78.904719, -2.907916) centre (-78.904719, -3.407916) ccw
  arc A202 (-92.404719, -16.407916) -> (-91.904719, -16.907916) centre (-91.904719, -16.407916) ccw
  arc A203 (-78.904719, -16.907916) -> (-78.404719, -16.407916) centre (-78.904719, -16.407916) ccw
  line L204 (-72.854719, -2.907916) -> (-59.854719, -2.907916)
  line L205 (-72.854719, -16.907916) -> (-59.854719, -16.907916)
  line L206 (-73.354719, -3.407916) -> (-73.354719, -16.407916)
  line L207 (-59.354719, -3.407916) -> (-59.354719, -16.407916)
  arc A204 (-72.854719, -2.907916) -> (-73.354719, -3.407916) centre (-72.854719, -3.407916) ccw
  arc A205 (-59.354719, -3.407916) -> (-59.854719, -2.907916) centre (-59.854719, -3.407916) ccw
  arc A206 (-73.354719, -16.407916) -> (-72.854719, -16.907916) centre (-72.854719, -16.407916) ccw
  arc A207 (-59.854719, -16.907916) -> (-59.354719, -16.407916) centre (-59.854719, -16.407916) ccw
  line L208 (-53.804719, -2.907916) -> (-40.804719, -2.907916)
  line L209 (-53.804719, -16.907916) -> (-40.804719, -16.907916)
  line L210 (-54.304719, -3.407916) -> (-54.304719, -16.407916)
  line L211 (-40.304719, -3.407916) -> (-40.304719, -16.407916)
  arc A208 (-53.804719, -2.907916) -> (-54.304719, -3.407916) centre (-53.804719, -3.407916) ccw
  arc A209 (-40.304719, -3.407916) -> (-40.804719, -2.907916) centre (-40.804719, -3.407916) ccw
  arc A210 (-54.304719, -16.407916) -> (-53.804719, -16.907916) centre (-53.804719, -16.407916) ccw
  arc A211 (-40.804719, -16.907916) -> (-40.304719, -16.407916) centre (-40.804719, -16.407916) ccw
  line L212 (-34.754719, -2.907916) -> (-21.754719, -2.907916)
  line L213 (-34.754719, -16.907916) -> (-21.754719, -16.907916)
  line L214 (-35.254719, -3.407916) -> (-35.254719, -16.407916)
  line L215 (-21.254719, -3.407916) -> (-21.254719, -16.407916)
  arc A212 (-34.754719, -2.907916) -> (-35.254719, -3.407916) centre (-34.754719, -3.407916) ccw
  arc A213 (-21.254719, -3.407916) -> (-21.754719, -2.907916) centre (-21.754719, -3.407916) ccw
  arc A214 (-35.254719, -16.407916) -> (-34.754719, -16.907916) centre (-34.754719, -16.407916) ccw
  arc A215 (-21.754719, -16.907916) -> (-21.254719, -16.407916) centre (-21.754719, -16.407916) ccw
  line L216 (-15.704719, -2.907916) -> (-2.704719, -2.907916)
  line L217 (-15.704719, -16.907916) -> (-2.704719, -16.907916)
  line L218 (-16.204719, -3.407916) -> (-16.204719, -16.407916)
  line L219 (-2.204719, -3.407916) -> (-2.204719, -16.407916)
  arc A216 (-15.704719, -2.907916) -> (-16.204719, -3.407916) centre (-15.704719, -3.407916) ccw
  arc A217 (-2.204719, -3.407916) -> (-2.704719, -2.907916) centre (-2.704719, -3.407916) ccw
  arc A218 (-16.204719, -16.407916) -> (-15.704719, -16.907916) centre (-15.704719, -16.407916) ccw
  arc A219 (-2.704719, -16.907916) -> (-2.204719, -16.407916) centre (-2.704719, -16.407916) ccw
  line L220 (3.345281, -2.907916) -> (16.345281, -2.907916)
  line L221 (3.345281, -16.907916) -> (16.345281, -16.907916)
  line L222 (2.845281, -3.407916) -> (2.845281, -16.407916)
  line L223 (16.845281, -3.407916) -> (16.845281, -16.407916)
  arc A220 (3.345281, -2.907916) -> (2.845281, -3.407916) centre (3.345281, -3.407916) ccw
  arc A221 (16.845281, -3.407916) -> (16.345281, -2.907916) centre (16.345281, -3.407916) ccw
  arc A222 (2.845281, -16.407916) -> (3.345281, -16.907916) centre (3.345281, -16.407916) ccw
  arc A223 (16.345281, -16.907916) -> (16.845281, -16.407916) centre (16.345281, -16.407916) ccw
  line L224 (22.395281, -2.907916) -> (35.395281, -2.907916)
  line L225 (22.395281, -16.907916) -> (35.395281, -16.907916)
  line L226 (21.895281, -3.407916) -> (21.895281, -16.407916)
  line L227 (35.895281, -3.407916) -> (35.895281, -16.407916)
  arc A224 (22.395281, -2.907916) -> (21.895281, -3.407916) centre (22.395281, -3.407916) ccw
  arc A225 (35.895281, -3.407916) -> (35.395281, -2.907916) centre (35.395281, -3.407916) ccw
  arc A226 (21.895281, -16.407916) -> (22.395281, -16.907916) centre (22.395281, -16.407916) ccw
  arc A227 (35.395281, -16.907916) -> (35.895281, -16.407916) centre (35.395281, -16.407916) ccw
  line L228 (41.445281, -2.907916) -> (54.445281, -2.907916)
  line L229 (41.445281, -16.907916) -> (54.445281, -16.907916)
  line L230 (40.945281, -3.407916) -> (40.945281, -16.407916)
  line L231 (54.945281, -3.407916) -> (54.945281, -16.407916)
  arc A228 (41.445281, -2.907916) -> (40.945281, -3.407916) centre (41.445281, -3.407916) ccw
  arc A229 (54.945281, -3.407916) -> (54.445281, -2.907916) centre (54.445281, -3.407916) ccw
  arc A230 (40.945281, -16.407916) -> (41.445281, -16.907916) centre (41.445281, -16.407916) ccw
  arc A231 (54.445281, -16.907916) -> (54.945281, -16.407916) centre (54.445281, -16.407916) ccw
  line L232 (60.495281, -2.907916) -> (73.495281, -2.907916)
  line L233 (60.495281, -16.907916) -> (73.495281, -16.907916)
  line L234 (59.995281, -3.407916) -> (59.995281, -16.407916)
  line L235 (73.995281, -3.407916) -> (73.995281, -16.407916)
  arc A232 (60.495281, -2.907916) -> (59.995281, -3.407916) centre (60.495281, -3.407916) ccw
  arc A233 (73.995281, -3.407916) -> (73.495281, -2.907916) centre (73.495281, -3.407916) ccw
  arc A234 (59.995281, -16.407916) -> (60.495281, -16.907916) centre (60.495281, -16.407916) ccw
  arc A235 (73.495281, -16.907916) -> (73.995281, -16.407916) centre (73.495281, -16.407916) ccw
  line L236 (86.689031, -2.907916) -> (99.689031, -2.907916)
  line L237 (86.689031, -16.907916) -> (99.689031, -16.907916)
  line L238 (86.189031, -3.407916) -> (86.189031, -16.407916)
  line L239 (100.189031, -3.407916) -> (100.189031, -16.407916)
  arc A236 (86.689031, -2.907916) -> (86.189031, -3.407916) centre (86.689031, -3.407916) ccw
  arc A237 (100.189031, -3.407916) -> (99.689031, -2.907916) centre (99.689031, -3.407916) ccw
  arc A238 (86.189031, -16.407916) -> (86.689031, -16.907916) centre (86.689031, -16.407916) ccw
  arc A239 (99.689031, -16.907916) -> (100.189031, -16.407916) centre (99.689031, -16.407916) ccw
  line L240 (112.882781, -2.907916) -> (125.882781, -2.907916)
  line L241 (112.882781, -16.907916) -> (125.882781, -16.907916)
  line L242 (112.382781, -3.407916) -> (112.382781, -16.407916)
  line L243 (126.382781, -3.407916) -> (126.382781, -16.407916)
  arc A240 (112.882781, -2.907916) -> (112.382781, -3.407916) centre (112.882781, -3.407916) ccw
  arc A241 (126.382781, -3.407916) -> (125.882781, -2.907916) centre (125.882781, -3.407916) ccw
  arc A242 (112.382781, -16.407916) -> (112.882781, -16.907916) centre (112.882781, -16.407916) ccw
  arc A243 (125.882781, -16.907916) -> (126.382781, -16.407916) centre (125.882781, -16.407916) ccw
  line L244 (131.932781, -2.907916) -> (144.932781, -2.907916)
  line L245 (131.932781, -16.907916) -> (144.932781, -16.907916)
  line L246 (131.432781, -3.407916) -> (131.432781, -16.407916)
  line L247 (145.432781, -3.407916) -> (145.432781, -16.407916)
  arc A244 (131.932781, -2.907916) -> (131.432781, -3.407916) centre (131.932781, -3.407916) ccw
  arc A245 (145.432781, -3.407916) -> (144.932781, -2.907916) centre (144.932781, -3.407916) ccw
  arc A246 (131.432781, -16.407916) -> (131.932781, -16.907916) centre (131.932781, -16.407916) ccw
  arc A247 (144.932781, -16.907916) -> (145.432781, -16.407916) centre (144.932781, -16.407916) ccw
  line L248 (-146.673469, -21.957916) -> (-133.673469, -21.957916)
  line L249 (-146.673469, -35.957916) -> (-133.673469, -35.957916)
  line L250 (-147.173469, -22.457916) -> (-147.173469, -35.457916)
  line L251 (-133.173469, -22.457916) -> (-133.173469, -35.457916)
  arc A248 (-146.673469, -21.957916) -> (-147.173469, -22.457916) centre (-146.673469, -22.457916) ccw
  arc A249 (-133.173469, -22.457916) -> (-133.673469, -21.957916) centre (-133.673469, -22.457916) ccw
  arc A250 (-147.173469, -35.457916) -> (-146.673469, -35.957916) centre (-146.673469, -35.457916) ccw
  arc A251 (-133.673469, -35.957916) -> (-133.173469, -35.457916) centre (-133.673469, -35.457916) ccw
  line L252 (-122.860969, -21.957916) -> (-109.860969, -21.957916)
  line L253 (-122.860969, -35.957916) -> (-109.860969, -35.957916)
  line L254 (-123.360969, -22.457916) -> (-123.360969, -35.457916)
  line L255 (-109.360969, -22.457916) -> (-109.360969, -35.457916)
  arc A252 (-122.860969, -21.957916) -> (-123.360969, -22.457916) centre (-122.860969, -22.457916) ccw
  arc A253 (-109.360969, -22.457916) -> (-109.860969, -21.957916) centre (-109.860969, -22.457916) ccw
  arc A254 (-123.360969, -35.457916) -> (-122.860969, -35.957916) centre (-122.860969, -35.457916) ccw
  arc A255 (-109.860969, -35.957916) -> (-109.360969, -35.457916) centre (-109.860969, -35.457916) ccw
  line L256 (-99.048469, -21.957916) -> (-86.048469, -21.957916)
  line L257 (-99.048469, -35.957916) -> (-86.048469, -35.957916)
  line L258 (-99.548469, -22.457916) -> (-99.548469, -35.457916)
  line L259 (-85.548469, -22.457916) -> (-85.548469, -35.457916)
  arc A256 (-99.048469, -21.957916) -> (-99.548469, -22.457916) centre (-99.048469, -22.457916) ccw
  arc A257 (-85.548469, -22.457916) -> (-86.048469, -21.957916) centre (-86.048469, -22.457916) ccw
  arc A258 (-99.548469, -35.457916) -> (-99.048469, -35.957916) centre (-99.048469, -35.457916) ccw
  arc A259 (-86.048469, -35.957916) -> (-85.548469, -35.457916) centre (-86.048469, -35.457916) ccw
  line L260 (-27.610969, -21.957916) -> (-14.610969, -21.957916)
  line L261 (-27.610969, -35.957916) -> (-14.610969, -35.957916)
  line L262 (-28.110969, -22.457916) -> (-28.110969, -35.457916)
  line L263 (-14.110969, -22.457916) -> (-14.110969, -35.457916)
  arc A260 (-27.610969, -21.957916) -> (-28.110969, -22.457916) centre (-27.610969, -22.457916) ccw
  arc A261 (-14.110969, -22.457916) -> (-14.610969, -21.957916) centre (-14.610969, -22.457916) ccw
  arc A262 (-28.110969, -35.457916) -> (-27.610969, -35.957916) centre (-27.610969, -35.457916) ccw
  arc A263 (-14.610969, -35.957916) -> (-14.110969, -35.457916) centre (-14.610969, -35.457916) ccw
  line L264 (43.826531, -21.957916) -> (56.826531, -21.957916)
  line L265 (43.826531, -35.957916) -> (56.826531, -35.957916)
  line L266 (43.326531, -22.457916) -> (43.326531, -35.457916)
  line L267 (57.326531, -22.457916) -> (57.326531, -35.457916)
  arc A264 (43.826531, -21.957916) -> (43.326531, -22.457916) centre (43.826531, -22.457916) ccw
  arc A265 (57.326531, -22.457916) -> (56.826531, -21.957916) centre (56.826531, -22.457916) ccw
  arc A266 (43.326531, -35.457916) -> (43.826531, -35.957916) centre (43.826531, -35.457916) ccw
  arc A267 (56.826531, -35.957916) -> (57.326531, -35.457916) centre (56.826531, -35.457916) ccw
  line L268 (67.639031, -21.957916) -> (80.639031, -21.957916)
  line L269 (67.639031, -35.957916) -> (80.639031, -35.957916)
  line L270 (67.139031, -22.457916) -> (67.139031, -35.457916)
  line L271 (81.139031, -22.457916) -> (81.139031, -35.457916)
  arc A268 (67.639031, -21.957916) -> (67.139031, -22.457916) centre (67.639031, -22.457916) ccw
  arc A269 (81.139031, -22.457916) -> (80.639031, -21.957916) centre (80.639031, -22.457916) ccw
  arc A270 (67.139031, -35.457916) -> (67.639031, -35.957916) centre (67.639031, -35.457916) ccw
  arc A271 (80.639031, -35.957916) -> (81.139031, -35.457916) centre (80.639031, -35.457916) ccw
  line L272 (93.832781, -21.957916) -> (106.832781, -21.957916)
  line L273 (93.832781, -35.957916) -> (106.832781, -35.957916)
  line L274 (93.332781, -22.457916) -> (93.332781, -35.457916)
  line L275 (107.332781, -22.457916) -> (107.332781, -35.457916)
  arc A272 (93.832781, -21.957916) -> (93.332781, -22.457916) centre (93.832781, -22.457916) ccw
  arc A273 (107.332781, -22.457916) -> (106.832781, -21.957916) centre (106.832781, -22.457916) ccw
  arc A274 (93.332781, -35.457916) -> (93.832781, -35.957916) centre (93.832781, -35.457916) ccw
  arc A275 (106.832781, -35.957916) -> (107.332781, -35.457916) centre (106.832781, -35.457916) ccw
  line L276 (112.882781, -21.957916) -> (125.882781, -21.957916)
  line L277 (112.882781, -35.957916) -> (125.882781, -35.957916)
  line L278 (112.382781, -22.457916) -> (112.382781, -35.457916)
  line L279 (126.382781, -22.457916) -> (126.382781, -35.457916)
  arc A276 (112.882781, -21.957916) -> (112.382781, -22.457916) centre (112.882781, -22.457916) ccw
  arc A277 (126.382781, -22.457916) -> (125.882781, -21.957916) centre (125.882781, -22.457916) ccw
  arc A278 (112.382781, -35.457916) -> (112.882781, -35.957916) centre (112.882781, -35.457916) ccw
  arc A279 (125.882781, -35.957916) -> (126.382781, -35.457916) centre (125.882781, -35.457916) ccw
  line L280 (131.932781, -21.957916) -> (144.932781, -21.957916)